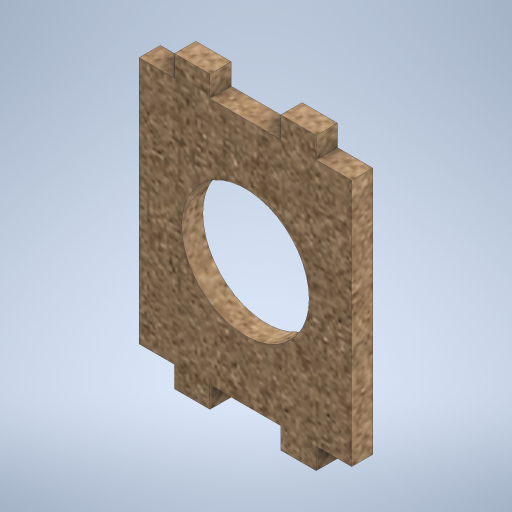
# Autodesk Inventor part: Sensor_Support
Saved by Autodesk Inventor 2024 (Build 280153000, 153)
## iProperties
Created: 2023-11-23
Part Number: Sensor_Support
Material: MDF Tablero de fibras de densidad media
Document SubType Name: Modeling
Designer: marco
Density: 0.8 g/cm^3
Appearance: Cartón - Ondulado
Author: marco
Autodesk Inventor part; units mm, degrees
ref_plane "YZ Plane" through (0, 0, 0) normal (1, 0, 0) x (0, 1, 0)
ref_plane "XZ Plane" through (0, 0, 0) normal (0, 1, 0) x (-1, 0, 0)
ref_plane "XY Plane" through (0, 0, 0) normal (0, 0, 1) x (1, 0, 0)
sketch "Boceto1" plane through (0, 0, 0) normal (0, 0, 1) x (1, 0, 0)
  circle A0 centre (0, 0) radius 9
  line L0 (15, -17.5) -> (15, 17.5)
  line L1 (15, 17.5) -> (10, 17.5)
  line L2 (10, 17.5) -> (10, 20.5)
  line L3 (10, 20.5) -> (5, 20.5)
  line L4 (5, 20.5) -> (5, 17.5)
  line L5 (5, 17.5) -> (-5, 17.5)
  line L6 (-5, 17.5) -> (-5, 20.5)
  line L7 (-5, 20.5) -> (-10, 20.5)
  line L8 (-10, 20.5) -> (-10, 17.5)
  line L9 (-10, 17.5) -> (-15, 17.5)
  line L10 (-15, 17.5) -> (-15, -17.5)
  line L11 (-15, -17.5) -> (-10, -17.5)
  line L12 (-10, -17.5) -> (-10, -20.5)
  line L13 (-10, -20.5) -> (-5, -20.5)
  line L14 (-5, -20.5) -> (-5, -17.5)
  line L15 (-5, -17.5) -> (5, -17.5)
  line L16 (5, -17.5) -> (5, -20.5)
  line L17 (5, -20.5) -> (10, -20.5)
  line L18 (10, -20.5) -> (10, -17.5)
  line L19 (10, -17.5) -> (15, -17.5)
  constraints: 40 end point, 1 centre point
extrude "Extrusión1" add sketch "Boceto1" along normal blind 3
